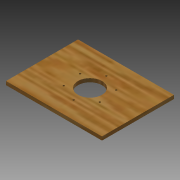
# Autodesk Inventor part: base_plate
Saved by Autodesk Inventor 2013 (Build 170138000, 138)
## iProperties
Created: 2014-10-12
Part Number: base_plate
Material: Plywood, Finish
Document SubType Name: Modeling
Designer: Masta
Density: 1 g/cm^3
Author: Masta
Autodesk Inventor part; units mm, degrees
ref_plane "YZ Plane" through (0, 0, 0) normal (1, 0, 0) x (0, 1, 0)
ref_plane "XZ Plane" through (0, 0, 0) normal (0, 1, 0) x (-1, 0, 0)
ref_plane "XY Plane" through (0, 0, 0) normal (0, 0, 1) x (1, 0, 0)
sketch "Sketch1" plane through (0, 0, 0) normal (0, 0, 1) x (1, 0, 0)
  line L0 (-80, -60) -> (80, -60)
  line L1 (80, -60) -> (80, 60)
  line L2 (80, 60) -> (-80, 60)
  line L3 (-80, 60) -> (-80, -60)
  line L4 (-80, -60) -> (80, 60) construction
  line L5 (80, -60) -> (-80, 60) construction
  circle A0 centre (0, 0) radius 20
  point P0 (25, 18.75)
  dimension "d0" = 160
  dimension "d1" = 120
  dimension "d2" = 40
  dimension "d5" = 25
  constraints: 12 end point, 2 midpoint, 2 parallel, 1 centre point, 1 coincident, 1 horizontal, 1 perpendicular, 1 point on line
  measures "d0" distance of L2.end L1.end
  measures "d1" distance of L1.end L0.end
  measures "d2" diameter of A0
  measures "d5" horizontal distance of point (0, 0) point (25, 18.75)
extrude "Extrusion1" add sketch "Sketch1" along normal blind 6
hole "Hole1" at (25, 18.75, 0) direction (0, 0, 1) diameter 3 end through all
pattern_circular "Circular Pattern1" count 6 over 360 about axis through (0, 0, 0) along (0, 0, 1) of "Hole1"
body "Solid1"
